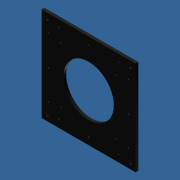
# Autodesk Inventor part: J002448
Saved by Autodesk Inventor 2015 SP1 (Build 190203100, 203)
## iProperties
Created: 2014-04-03
Material: ALUMINUM, 6061-T651
Vendor: HHMI: JFRC - ID&F
Document SubType Name: Modeling
Designer: NEGRASHOVI
Mass: 3185.65 g
Surface Area: 2012.9 cm^2
Volume: 1179.87 cm^3
Density: 2.7 g/cm^3
Part Number: J002448
Description: ARENA SUPPORT
Project: P-159707
Appearance: Glossy - Black
RuleStatus: InUse
AfterDocSave0: file://Part Number Cleaner
LAB/DEPT: RUBIN (LAB)
REQUESTING SCIENTIST: ASO, YOSHI
SURFACE ROUGHNESS: 32 ra
DESIGN DEPARTMENT: HHMI: JRC - ID&F
SPECIAL FINISH: ANODIZE PER MIL-A-8625F, TYPE II, CLASS 2 (BLACK)
ALTERED ITEM PART NUMBER: N/A
ALTERED ITEM VENDOR: N/A
ALTERED ITEM DESCRIPTION: N/A
Author: NEGRASHOVI
Revision Number: B
Autodesk Inventor part; units mm, degrees
ref_plane "YZ Plane" through (0, 0, 0) normal (1, 0, 0) x (0, 1, 0)
ref_plane "XZ Plane" through (0, 0, 0) normal (0, 1, 0) x (-1, 0, 0)
ref_plane "XY Plane" through (0, 0, 0) normal (0, 0, 1) x (1, 0, 0)
sketch "Sketch1" plane through (0, 0, 0) normal (0, 0, 1) x (1, 0, 0)
  line L0 (-107.95, -107.95) -> (107.95, -107.95)
  line L1 (107.95, -107.95) -> (107.95, 107.95)
  line L2 (107.95, 107.95) -> (-107.95, 107.95)
  line L3 (-107.95, 107.95) -> (-107.95, -107.95)
  line L4 (-107.95, -107.95) -> (107.95, 107.95) construction
  point P0 (0, 0)
  point P1 (0, 0)
  dimension "d0" = 215.9
  dimension "d1" = 215.9
  constraints: 10 end point, 2 parallel, 1 coincident, 1 horizontal, 1 midpoint, 1 perpendicular
  measures "d0" distance of L1.end L2.end
  measures "d1" distance of L0.end L1.end
extrude "Extrusion1" add sketch "Sketch1" along normal blind 6.35
sketch "Sketch3" plane through (0, 0, 6.35) normal (0, 0, 1) x (1, 0, 0)
  circle A0 centre (0, 0) radius 57.785
  dimension "d44" = 115.57
  constraints: 1 centre point, 1 coincident
  measures "d44" diameter of A0
extrude "Extrusion3" cut sketch "Sketch3" against normal through all
sketch "Sketch5" plane through (0, 0, 6.35) normal (0, 0, 1) x (1, 0, 0)
  line L0 (-95.25, -95.25) -> (95.25, -95.25) construction
  line L1 (95.25, -95.25) -> (95.25, 95.25) construction
  line L2 (95.25, 95.25) -> (-95.25, 95.25) construction
  line L3 (-95.25, 95.25) -> (-95.25, -95.25) construction
  line L4 (-95.25, -95.25) -> (95.25, 95.25) construction
  point P0 (0, 0)
  point P1 (0, 0)
  point P2 (0, 0)
  dimension "d15" = 190.5
  dimension "d16" = 190.5
  constraints: 10 end point, 6 coincident, 2 parallel, 1 horizontal, 1 midpoint, 1 perpendicular
  measures "d15" distance of L0.end L1.end
  measures "d16" distance of L1.end L2.end
hole "Hole1" at (-95.25, 95.25, 6.35) at (95.25, 95.25, 6.35) at (95.25, -95.25, 6.35) at (-95.25, -95.25, 6.35) direction (0, 0, -1) diameter 4.4958 end through all counterbore diameter 7.9502 counterbore depth 4.1656 clearance for "Socket Head Cap Screw" size "#8" standard "Ansi Unified Screw Threads"
sketch "Sketch6" plane through (0, 0, 0) normal (0, 0, -1) x (-1, 0, 0)
  line L0 (-63.5, -63.5) -> (63.5, -63.5) construction
  line L1 (63.5, -63.5) -> (63.5, 63.5) construction
  line L2 (63.5, 63.5) -> (-63.5, 63.5) construction
  line L3 (-63.5, 63.5) -> (-63.5, -63.5) construction
  line L4 (-63.5, -63.5) -> (63.5, 63.5) construction
  point P0 (0, 0)
  point P1 (0, 0)
  dimension "d24" = 127
  dimension "d25" = 127
  constraints: 10 end point, 5 coincident, 2 parallel, 1 horizontal, 1 midpoint, 1 perpendicular
  measures "d24" distance of L1.end L2.end
  measures "d25" distance of L0.end L1.end
hole "Hole2" at (63.5, 63.5, 0) at (-63.5, 63.5, 0) at (-63.5, -63.5, 0) at (63.5, -63.5, 0) direction (0, 0, 1) diameter 3.302 end through all thread size "8-32 UNC" class "2B" standard "ANSI Unified Screw Threads"
sketch "Sketch7" plane through (0, 0, 6.35) normal (0, 0, 1) x (1, 0, 0)
  line L0 (-91.44, -91.44) -> (91.44, -91.44) construction
  line L1 (91.44, -91.44) -> (91.44, 91.44) construction
  line L2 (91.44, 91.44) -> (-91.44, 91.44) construction
  line L3 (-91.44, 91.44) -> (-91.44, -91.44) construction
  line L4 (-91.44, -91.44) -> (91.44, 91.44) construction
  line L5 (-151.13, 0) -> (151.13, 0) construction
  line L6 (0, -151.13) -> (0, 151.13) construction
  point P0 (0, 0)
  point P1 (0, 0)
  point P2 (-68.58, 91.44)
  point P3 (0, 91.44)
  point P4 (68.58, 91.44)
  point P5 (91.44, 68.58)
  point P6 (91.44, 0)
  point P7 (91.44, -68.58)
  point P8 (68.58, -91.44)
  point P9 (0, -91.44)
  point P10 (-68.58, -91.44)
  point P11 (-91.44, -68.58)
  point P12 (-91.44, 0)
  point P13 (-91.44, 68.58)
  dimension "d33" = 182.88
  dimension "d34" = 182.88
  dimension "d35" = 22.86
  dimension "d36" = 22.86
  constraints: 12 point on line, 10 end point, 6 symmetric about line, 5 midpoint, 2 parallel, 1 coincident, 1 horizontal, 1 perpendicular
  measures "d33" distance of L1.end L2.end
  measures "d34" distance of L0.end L1.end
  measures "d35" distance from line of point (-91.44, 68.58) L2
  measures "d36" distance from line of point (-68.58, 91.44) L3
hole "Hole3" at (-68.58, 91.44, 6.35) at (0, 91.44, 6.35) at (68.58, 91.44, 6.35) at (91.44, 68.58, 6.35) at (91.44, 0, 6.35) at (91.44, -68.58, 6.35) at (68.58, -91.44, 6.35) at (0, -91.44, 6.35) at (-68.58, -91.44, 6.35) at (-91.44, -68.58, 6.35) at (-91.44, 0, 6.35) at (-91.44, 68.58, 6.35) direction (0, 0, -1) diameter 3.302 end through all thread size "8-32 UNC" class "2B" standard "ANSI Unified Screw Threads"
equation "\"d15\" = d16"
equation "\"d25\" = d24"
body "Solid1"
